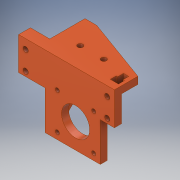
# Autodesk Inventor part: Hopper Motor Holder
Saved by Autodesk Inventor 2018 (Build 220112000, 112)
## iProperties
Created: 2013-10-17
Part Number: Hopper Motor Holder
Material: ABS Plastic
Document SubType Name: Modeling
Designer: Gabriel Smolnycki
Mass: 42.8038 g
Surface Area: 160.409 cm^2
Volume: 40.3809 cm^3
Density: 1.06 g/cm^3
Appearance: Smooth - Light Orange
Sending System: SolidWorks 2017
Last Author: Gabriel Smolnycki
Last Saved: 2017-09-14
Author: Gabriel Smolnycki
Autodesk Inventor part; units mm, degrees
ref_plane "YZ Plane" through (0, 0, 0) normal (1, 0, 0) x (0, 1, 0)
ref_plane "XY Plane" through (0, 0, 0) normal (0, 0, 1) x (1, 0, 0)
ref_plane "Work Plane1" through (0, -33, 0) normal (0, 1, 0) x (-1, 0, 0)
sketch "Sketch1" plane through (0, -33, 0) normal (0, 1, 0) x (-1, 0, 0)
  line L0 (-65, -10) -> (-65, 10)
  line L1 (16.5, -30) -> (16.5, 10)
  line L2 (16.5, 10) -> (-65, 10)
  line L3 (-10, -30) -> (-65, -10)
  line L4 (16.5, -30) -> (-10, -30)
  constraints: 10 end point, 2 horizontal, 2 vertical
extrude "Extrusion7" add sketch "Sketch1" along normal blind 61
sketch "Sketch2" plane through (65, -33, 10) normal (1, 0, 0) x (0, 0, -1)
  line L0 (6, 0) -> (40, 0)
  line L1 (40, 55) -> (40, 0)
  line L2 (6, 0) -> (6, 55)
  line L3 (40, 55) -> (6, 55)
  constraints: 8 end point, 2 horizontal, 2 vertical
extrude "Extrusion6" cut sketch "Sketch2" against normal blind 55
sketch "Sketch3" plane through (65, -33, 10) normal (1, 0, 0) x (0, 0, -1)
  line L0 (0, 33) -> (6, 33)
  line L1 (0, 0) -> (6, 0)
  line L2 (6, 0) -> (6, 33)
  line L3 (0, 0) -> (0, 33)
  constraints: 8 end point, 2 horizontal, 2 vertical
extrude "Extrusion5" cut sketch "Sketch3" against normal blind 12
sketch "Sketch4" plane through (-16.5, -33, -30) normal (-1, 0, 0) x (0, 0, 1)
  line L0 (0, 0) -> (40, 0)
  line L1 (0, 33) -> (0, 0)
  line L2 (40, 33) -> (0, 33)
  line L3 (40, 0) -> (40, 33)
  constraints: 8 end point, 2 horizontal, 2 vertical
extrude "Extrusion4" cut sketch "Sketch4" against normal blind 22.5
sketch "Sketch5" plane through (65, 22, 4) normal (0, 0, -1) x (-1, 0, 0)
  line L0 (9.5, 0) -> (2.5, 0)
  line L1 (9.5, 6) -> (2.5, 6)
  line L2 (9.5, 6) -> (9.5, 0)
  line L3 (2.5, 6) -> (2.5, 0)
  constraints: 8 end point, 2 horizontal, 2 vertical
extrude "Extrusion3" cut sketch "Sketch5" along normal blind 5
sketch "Sketch6" plane through (10, 28, -30) normal (0, 0, -1) x (-1, 0, 0)
  line L0 (10, 0) -> (26.5, 0)
  line L1 (26.5, 0) -> (26.5, -28)
  line L2 (10, -28) -> (26.5, -28)
  line L3 (10, 0) -> (10, -28)
  constraints: 8 end point, 2 horizontal, 2 vertical
extrude "Extrusion2" cut sketch "Sketch6" against normal blind 30
sketch "Sketch7" plane through (65, 22, -1) normal (0, 0, 1) x (1, 0, 0)
  line L0 (-8.25, 0) -> (-3.75, 0)
  line L1 (-3.75, 6) -> (-3.75, 0)
  line L2 (-8.25, 6) -> (-8.25, 0)
  line L3 (-8.25, 6) -> (-3.75, 6)
  constraints: 8 end point, 2 horizontal, 2 vertical
extrude "Extrusion1" cut sketch "Sketch7" against normal blind 5 draft 0
chamfer "Chamfer1" distance 34 distance2 33 1 edges at (8, -33, -30) measured on face at (8, -33, -29.5)
hole "Hole12" at (38, 22, -8) direction (0, 1, 0) diameter 4.5 depth 6 tip angle 118
hole "Hole11" at (18, 22, -8) direction (0, 1, 0) diameter 4.5 depth 6 tip angle 118
hole "Hole10" at (10, 17.5, -24) direction (-1, 0, 0) diameter 4.5 depth 10 tip angle 118
hole "Hole9" at (59, 20, 10) direction (0, 0, -1) diameter 4.5 depth 6 tip angle 118
hole "Hole8" at (59, 4, 10) direction (0, 0, -1) diameter 4.5 depth 6 tip angle 118
hole "Hole7" at (-10.5, 20, 10) direction (0, 0, -1) diameter 4.5 depth 10 tip angle 118
sketch "Sketch13" plane through (-16.5, 28, 10) normal (0, 0, 1) x (1, 0, 0)
  point P0 (6, -8)
hole "Hole6" at (47.5, 3.5, 4) direction (0, 0, 1) diameter 3.5 depth 6 tip angle 118
sketch "Sketch12" plane through (-16.5, 28, 10) normal (0, 0, 1) x (1, 0, 0)
  point P0 (75.5, -24)
hole "Hole5" at (47.5, -27.5, 4) direction (0, 0, 1) diameter 3.5 depth 6 tip angle 118
sketch "Sketch11" plane through (-16.5, 28, 10) normal (0, 0, 1) x (1, 0, 0)
  point P0 (75.5, -8)
hole "Hole4" at (16.5, -27.5, 4) direction (0, 0, 1) diameter 3.5 depth 6 tip angle 118
sketch "Sketch10" plane through (10, -33, 10) normal (1, 0, 0) x (0, 0, -1)
  point P0 (34, 50.5)
hole "Hole3" at (16.5, 3.5, 4) direction (0, 0, 1) diameter 3.5 depth 6 tip angle 118
sketch "Sketch9" plane through (65, 22, -10) normal (0, -1, 0) x (1, 0, 0)
  point P0 (-47, 2)
hole "Hole2" at (32, -12, 4) direction (0, 0, 1) diameter 24 depth 6 tip angle 118
sketch "Sketch8" plane through (65, 22, -10) normal (0, -1, 0) x (1, 0, 0)
  point P0 (-27, 2)
hole "Hole1" at (-10.5, 4, 10) direction (0, 0, -1) diameter 4.5 depth 10 tip angle 118
sketch "Sketch14" plane through (65, 0, 4) normal (0, 0, -1) x (-1, 0, 0)
  point P0 (17.5, 3.5)
sketch "Sketch15" plane through (65, 0, 4) normal (0, 0, -1) x (-1, 0, 0)
  point P0 (17.5, -27.5)
sketch "Sketch16" plane through (65, 0, 4) normal (0, 0, -1) x (-1, 0, 0)
  point P0 (48.5, -27.5)
sketch "Sketch17" plane through (65, 0, 4) normal (0, 0, -1) x (-1, 0, 0)
  point P0 (48.5, 3.5)
sketch "Sketch18" plane through (65, 0, 4) normal (0, 0, -1) x (-1, 0, 0)
  point P0 (33, -12)
sketch "Sketch19" plane through (-16.5, 28, 10) normal (0, 0, 1) x (1, 0, 0)
  point P0 (6, -24)
body "Solid3"
